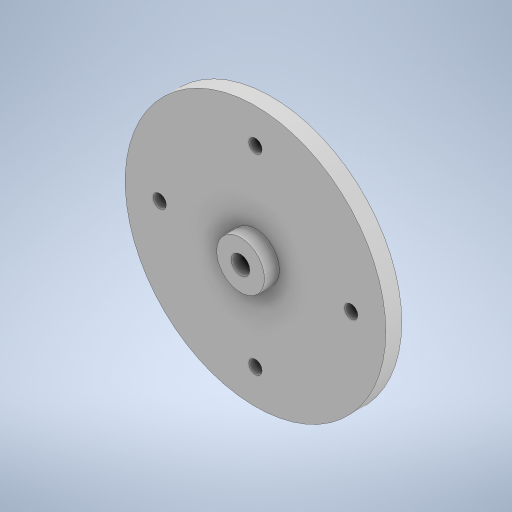
# Autodesk Inventor part: 좌측 축
Saved by Autodesk Inventor 2023.1 (Build 271208000, 208)
## iProperties
Created: 2022-08-13
Part Number: 좌측 축
Material: 일반
Document SubType Name: Modeling
Designer: fly01
Density: 1 g/cm^3
Appearance: 기본값
Author: fly01
Autodesk Inventor part; units mm, degrees
ref_plane "YZ Plane" through (0, 0, 0) normal (1, 0, 0) x (0, 1, 0)
ref_plane "XZ Plane" through (0, 0, 0) normal (0, 1, 0) x (-1, 0, 0)
ref_plane "XY Plane" through (0, 0, 0) normal (0, 0, 1) x (1, 0, 0)
sketch "스케치1" plane through (0, 0, 0) normal (0, 0, 1) x (1, 0, 0)
  circle A0 centre (0, 0) radius 24.5
  circle A1 centre (0, 0) radius 4.5
  circle A2 centre (0, 0) radius 1.75
  circle A3 centre (0, 18) radius 1.25
  circle A4 centre (-18, 0) radius 1.25
  circle A5 centre (0, -18) radius 1.25
  circle A6 centre (18, 0) radius 1.25
  dimension "d0" = 49
  dimension "d1" = 9
  dimension "d2" = 3.5
  dimension "d7" = 2.5
  dimension "d8" = 18
  dimension "d11" = 360
  constraints: 7 centre point, 3 coincident, 9 other
  measures "d0" diameter of A0
  measures "d1" diameter of A1
  measures "d2" diameter of A2
  measures "d7" diameter of A3
  measures "d8" distance of point (0, 0) A3.centre
extrude "돌출1" add sketch "스케치1" against normal blind 3 contours A0 | A1
extrude "돌출2" add sketch "스케치1" along normal blind 2.8 contours A1
sketch "스케치2" plane through (0, 0, -3) normal (0, 0, -1) x (-1, 0, 0)
  circle A0 centre (0, 0) radius 3
  dimension "d13" = 6
  constraints: 1 centre point, 1 coincident
  measures "d13" diameter of A0
extrude "돌출3" cut sketch "스케치2" against normal blind 2
